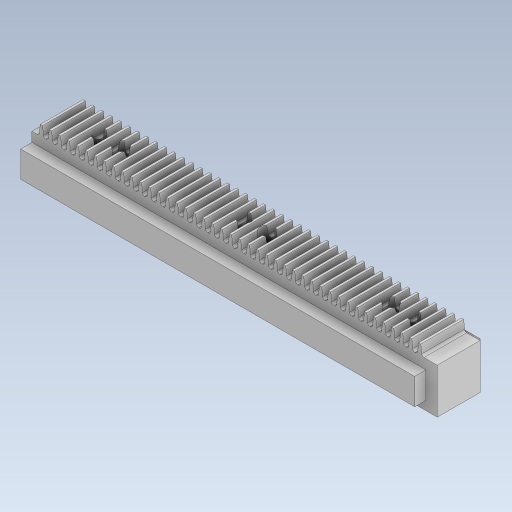
# Autodesk Inventor part: Rack Lifter 2
Saved by Autodesk Inventor 2023.5 (Build 275446000, 446)
## iProperties
Created: 2025-09-06
Part Number: Rack Lifter 2
Material: Generic
Document SubType Name: Modeling
Designer: Guntur
Density: 1 g/cm^3
Appearance: Default
Author: Guntur
## iProperties of the stored document Rack Lifter 2_3DPrint.ipt
Created: 2025-09-06
Part Number: Rack Lifter 2_3DPrint
Material: Generic
Document SubType Name: Modeling
Designer: Guntur
Density: 1 g/cm^3
Appearance: Default
Author: Guntur
Autodesk Inventor part; units mm, degrees
ref_plane "YZ Plane" through (0, 0, 0) normal (1, 0, 0) x (0, 1, 0)
sketch "Sketch1" plane through (0, 0, 0) normal (0, 1, 0) x (-1, 0, 0)
  line L0 (50, 9.5) -> (-50, 9.5)
  line L1 (-50, 9.5) -> (-50, -9.5)
  line L2 (-50, -9.5) -> (50, -9.5)
  line L3 (50, -9.5) -> (50, 9.5)
  line L4 (50, 9.5) -> (-50, -9.5) construction
  line L5 (-50, 9.5) -> (50, -9.5) construction
  line L6 (-50, 9.5) -> (-45, 9.5)
  line L7 (-45, 9.5) -> (-45, 4.5)
  line L8 (-45, 4.5) -> (-50, 4.5)
  line L9 (-50, 4.5) -> (-50, 9.5)
  line L10 (-50, -9.5) -> (-45, -9.5)
  line L11 (-45, -9.5) -> (-45, -4.5)
  line L12 (-45, -4.5) -> (-50, -4.5)
  line L13 (-50, -4.5) -> (-50, -9.5)
  point P0 (0, 0)
  point P1 (-45, 9.5)
  dimension "d0" = 100
  dimension "d1" = 19
  dimension "d2" = 5
  dimension "d3" = 5
  dimension "d4" = 5
  dimension "d5" = 5
  constraints: 28 end point, 6 parallel, 3 horizontal, 3 perpendicular, 2 midpoint
  measures "d0" distance of L2.end L1.end
  measures "d1" distance of L1.end L0.end
  measures "d2" distance of L7.end L8.end
  measures "d3" distance of L6.end L7.end
  measures "d4" distance of L12.end L11.end
  measures "d5" distance of L11.end L10.end
extrude "Extrusion1" add sketch "Sketch1" along normal blind 20 contours L3 L2 L11 L12 L1 L8 L7 L0
sketch "Sketch3" plane through (-50, 0, 9.5) normal (0, 0, 1) x (1, 0, 0)
  line L0 (100, 0) -> (100, 20) projected
  line L1 (0, 4) -> (100, 4)
  line L2 (100, 4) -> (100, 15.7)
  line L3 (100, 15.7) -> (0, 15.7)
  line L4 (0, 15.7) -> (0, 4)
  line L5 (0, 4) -> (100, 15.7) construction
  line L6 (100, 4) -> (0, 15.7) construction
  line L7 (95, 0) -> (95, 20) projected
  line L8 (95, 4) -> (95, 15.7)
  point P0 (50, 0)
  point P1 (50, 9.85)
  dimension "d8" = 11.7
  constraints: 14 end point, 5 point on line, 2 midpoint, 2 parallel, 1 horizontal, 1 perpendicular
  measures "d8" distance of L2.end L1.end
extrude "Extrusion2" add sketch "Sketch3" along normal blind 5 contours L1 L4 L3 L7
sketch "Sketch4" plane through (45, 0, -9.5) normal (0, 0, -1) x (-1, 0, 0)
  line L0 (-5, 0) -> (-5, 20) projected
  line L1 (95, 15.7) -> (-5, 15.7)
  line L2 (-5, 15.7) -> (-5, 4)
  line L3 (-5, 4) -> (95, 4)
  line L4 (95, 4) -> (95, 15.7)
  line L5 (95, 15.7) -> (-5, 4) construction
  line L6 (-5, 15.7) -> (95, 4) construction
  line L7 (0, 15.7) -> (0, 20) projected
  line L8 (0, 15.7) -> (0, 4.585)
  line L9 (0, 0) -> (0, 20) projected
  line L10 (0, 4) -> (0, 4.6)
  point P0 (45, 0)
  point P1 (45, 9.85)
  point P2 (-5, 15.7)
  dimension "d11" = 11.7
  constraints: 16 end point, 5 point on line, 2 midpoint, 2 parallel, 2 perpendicular, 1 horizontal
  measures "d11" distance of L2.end L1.end
extrude "Extrusion3" add sketch "Sketch4" along normal blind 5
ref_plane "Work Plane1" through (45, 0, 0) normal (0, 0, -1) x (-1, 0, 0)
sketch "Sketch7" plane through (45, 0, 0) normal (0, 0, -1) x (-1, 0, 0)
  line L0 (0, 22) -> (95, 22)
  line L1 (0, 24.5) -> (95, 24.5)
  line L2 (0, 22) -> (2, 22)
  line L3 (2.785, 25.4) -> (2.785, 18.6261) construction
  line L4 (0, 30) -> (0, 24.5)
  line L5 (0, 0) -> (0, 20) projected
  line L6 (95, 20) -> (0, 20) projected
  line L7 (0, 20) -> (95, 20)
  arc A0 (2.285, 24.5) -> (1.835, 20) centre (74.1604, 15.04) ccw
  arc A1 (3.735, 20) -> (3.285, 24.5) centre (-68.5904, 15.04) ccw
  point P0 (45, 0)
  point P1 (3.57, 22)
  point P2 (3.285, 24.5)
  point P3 (1.835, 20)
  point P4 (3.735, 20)
  dimension "d27" = 95
  dimension "d28" = 1
  dimension "d29" = 1.9
  constraints: 12 end point, 5 point on circle, 4 point on line, 3 symmetric about line, 2 centre point, 2 horizontal, 2 vertical, 1 coincident, 1 collinear, 1 horizontal alignment, 3 other
  measures "d27" distance of L5.end L6.start
  measures "d28" distance of A1.end A0.start
  measures "d29" distance of A1.start A0.end
extrude "Extrusion5" add sketch "Sketch7" along normal blind 9.5 and the other way blind 9.5
fillet "Fillet1" radius 1 2 edges at (43.165, 20, 0) (41.265, 20, 0)
extrude "Extrusion7" add sketch "Sketch1" along normal blind 20 contours L7 L8 L1 L0 | L2 L1 L12 L11
sketch "Sketch10" plane through (-50, 0, -9.5) normal (-1, 0, 0) x (0, 0, 1)
  line L0 (24, 4) -> (24, 15.7) projected
  line L1 (24, 15.7) -> (24, 4)
  line L2 (19, 4) -> (24, 4) projected
  line L3 (24, 4) -> (19, 4)
  line L4 (19, 4) -> (19, 0)
  line L5 (19, 0) -> (0, 0)
  line L6 (0, 4) -> (-5, 4) projected
  line L7 (0, 0) -> (0, 4)
  line L8 (0, 4) -> (-5, 4)
  line L9 (0, 15.7) -> (-5, 15.7) projected
  line L10 (-5, 4) -> (-5, 15.7)
  line L11 (-5, 15.7) -> (0, 15.7)
  line L12 (0, 15.7) -> (0, 20) projected
  line L13 (0, 15.7) -> (0, 20)
  line L14 (19, 20) -> (19, 20.9189) projected
  line L15 (0, 20) -> (19, 20)
  line L16 (19, 20) -> (19, 15.7)
  line L17 (19, 15.7) -> (24, 15.7) projected
  line L18 (19, 15.7) -> (24, 15.7)
  point P0 (9.5, 0)
  constraints: 24 end point, 7 perpendicular, 4 collinear, 1 vertical
extrude "Extrusion9" add sketch "Sketch10" along normal blind 80
pattern_linear "Rectangular Pattern2" count 43 spacing 4 along (-1, 0, 0) of "Extrusion5", "Fillet1"
sketch "Sketch11" plane through (0, 0, 0) normal (0, -1, 0) x (1, 0, 0)
  circle A0 centre (30, 0) radius 1.5
  line L0 (50, 9.5) -> (50, -9.5) projected
  circle A1 centre (20, 0) radius 1.5
  circle A2 centre (-110, 0) radius 1.5
  line L1 (-130, -9.5) -> (-130, 9.5) projected
  circle A3 centre (-100, 0) radius 1.5
  line L2 (-130, 9.5) -> (50, 9.5) projected
  line L3 (-40, 9.5) -> (-40, -9.5)
  line L4 (50, -9.5) -> (-130, -9.5) projected
  circle A4 centre (-35, 0) radius 1.5
  circle A5 centre (-45, 0) radius 1.5
  point P0 (0, 0)
  dimension "d60" = 3
  dimension "d61" = 20
  dimension "d62" = 3
  dimension "d63" = 10
  dimension "d64" = 3
  dimension "d65" = 20
  dimension "d66" = 3
  dimension "d67" = 10
  dimension "d68" = 3
  dimension "d69" = 5
  constraints: 6 centre point, 2 end point, 2 midpoint, 1 symmetric about line, 1 other
  measures "d60" diameter of A0
  measures "d61" distance from line of L0 A0.centre
  measures "d62" diameter of A1
  measures "d63" distance of A0.centre A1.centre
  measures "d64" diameter of A2
  measures "d65" distance from line of L1 A2.centre
  measures "d66" diameter of A3
  measures "d67" distance of A3.centre A2.centre
  measures "d68" diameter of A4
  measures "d69" distance from line of L3 A4.centre
extrude "Extrusion10" cut sketch "Sketch11" against normal blind 30 contours A0 | A1 | A2 | A3 | A4 | A5
ref_plane "Work Plane3" through (45, 9.85, 14.5) normal (0, 1, 0) x (1, 0, 0)
sketch "Sketch12" plane through (45, 9.85, 14.5) normal (0, 1, 0) x (1, 0, 0)
  circle A0 centre (-155, 14.5) radius 1.5 projected
  circle A1 centre (-155, 14.5) radius 3
  circle A2 centre (-145, 14.5) radius 1.5 projected
  circle A3 centre (-145, 14.5) radius 3
  circle A4 centre (-90, 14.5) radius 1.5 projected
  circle A5 centre (-90, 14.5) radius 3
  circle A6 centre (-80, 14.5) radius 1.5 projected
  circle A7 centre (-80, 14.5) radius 3
  arc A8 (-26.285, 15.2738) -> (-26.285, 13.7262) centre (-25, 14.5) ccw projected
  circle A9 centre (-25, 14.5) radius 3
  circle A10 centre (-15, 14.5) radius 1.5 projected
  circle A11 centre (-15, 14.5) radius 2.5
  point P0 (-45, 14.5)
  dimension "d72" = 6
  dimension "d73" = 6
  dimension "d74" = 6
  dimension "d75" = 6
  dimension "d76" = 6
  dimension "d77" = 5
  constraints: 6 centre point, 6 coincident
  measures "d72" diameter of A1
  measures "d73" diameter of A3
  measures "d74" diameter of A5
  measures "d75" diameter of A7
  measures "d76" diameter of A9
  measures "d77" diameter of A11
extrude "Extrusion11" cut sketch "Sketch12" along normal blind 15 contours A0 | A1 | A3 | A4 | A5 | A6 | A7 | A9 | A11
sketch "Sketch13" plane through (50, 0, 9.5) normal (1, 0, 0) x (0, 0, -1)
  line L0 (24, 4) -> (19, 4) projected
  line L1 (19, 15.7) -> (24, 15.7) projected
  line L2 (24, 4) -> (19, 4)
  line L3 (19, 4) -> (19, 15.7)
  line L4 (19, 15.7) -> (24, 15.7)
  line L5 (24, 15.7) -> (24, 4)
  point P0 (9.5, 0)
  constraints: 8 end point, 2 parallel, 1 horizontal, 1 perpendicular
extrude "Extrusion12" cut sketch "Sketch13" against normal blind 5
body "Solid1"
